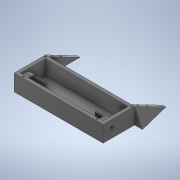
# Autodesk Inventor part: BodyWedgeV2
Saved by Autodesk Inventor 2020 (Build 240168000, 168)
## iProperties
Created: 2023-11-26
Part Number: BodyWedgeV2
Material: Thermoplastic Resin
Document SubType Name: Modeling
Designer: smz3rm
Density: 1.28 g/cm^3
Appearance: Smooth - Black
Mass: 160.779 g
Surface Area: 550.201 cm^2
Volume: 125.609 cm^3
Author: smz3rm
Autodesk Inventor part; units mm, degrees
ref_plane "YZ Plane" through (0, 0, 0) normal (1, 0, 0) x (0, 1, 0)
ref_plane "XZ Plane" through (0, 0, 0) normal (0, 1, 0) x (-1, 0, 0)
sketch "Sketch1" plane through (0, 0, 0) normal (0, 1, 0) x (-1, 0, 0)
  line L0 (85, 30) -> (-85, 30)
  line L1 (-85, 30) -> (-85, -30)
  line L2 (-85, -30) -> (85, -30)
  line L3 (85, -30) -> (85, 30)
  line L4 (85, 30) -> (-85, -30) construction
  line L5 (-85, 30) -> (85, -30) construction
  line L6 (0, -42) -> (0, 42) projected
  point P0 (0, 0)
  point P1 (-100, -30)
  point P2 (-85, -27)
  dimension "d0" = 170
  dimension "d1" = 60
  dimension "d32" = 15
  constraints: 12 end point, 2 midpoint, 2 parallel, 2 point on line, 1 horizontal, 1 perpendicular
  measures "d0" distance of L2.end L1.end
  measures "d1" distance of L1.end L0.end
  measures "d32" distance of L1.end point (-100, -30)
extrude "Extrusion1" add sketch "Sketch1" along normal blind 3
sketch "Sketch2" plane through (0, 3, 0) normal (0, 1, 0) x (1, 0, 0)
  line L0 (-85, 30) -> (-85, -30) projected
  line L1 (-85, -30) -> (85, -30) projected
  line L2 (85, -30) -> (85, 30) projected
  line L3 (79, -24) -> (-79, -24)
  line L4 (-79, -24) -> (-79, 24)
  line L5 (-79, 24) -> (79, 24)
  line L6 (79, 24) -> (79, -24)
  line L7 (79, -24) -> (-79, 24) construction
  line L8 (-79, -24) -> (79, 24) construction
  line L9 (85, 30) -> (-85, 30) projected
  point P0 (0, 0)
  dimension "d36" = 158
  dimension "d37" = 48
  constraints: 12 end point, 2 midpoint, 2 parallel, 1 horizontal, 1 perpendicular
  measures "d36" distance of L4.end L5.end
  measures "d37" distance between parallel lines of L5 L3
extrude "Extrusion2" add sketch "Sketch2" along normal blind 28
sketch "Sketch7" plane through (-79, 3, 24) normal (1, 0, 0) x (0, 0, -1)
  circle A0 centre (10, 14) radius 8
  line L0 (54, -3) -> (-6, -3) projected
  circle A1 centre (10, 14) radius 10
  line L1 (0, 14) -> (0, 0)
  line L2 (0, 14) -> (20, 14)
  line L3 (20, 14) -> (20, 0)
  line L4 (-6, -3) -> (-6, 28) projected
  line L5 (0, 0) -> (20, 0)
  line L6 (10, 24) -> (0, 24)
  line L7 (0, 0) -> (0, 28) projected
  line L8 (0, 14) -> (0, 24)
  point P0 (24, -3)
  point P1 (54, -3)
  dimension "MotorDiameter" = 16
  dimension "d18" = 17
  dimension "d20" = 2
  dimension "d40" = 20
  dimension "d62" = 10
  constraints: 12 end point, 3 horizontal, 3 point on circle, 2 centre point, 2 vertical, 1 perpendicular, 1 point on line
  measures "MotorDiameter" diameter of A0
  measures "d18" distance from line of L0 A0.centre
  measures "d20" radial gap between concentric circles of A0 A1
  measures "d40" distance between parallel lines of L3 L1
  measures "d62" distance of L6.start L6.end
extrude "Extrusion5" add sketch "Sketch7" along normal blind 11.25 contours L2 A1 A0 | A0 L2 A1 | L3 L5 L1 A1 | L7 L6 A1
sketch "Sketch8" plane through (-67.75, 3, 24) normal (1, 0, 0) x (0, 0, -1)
  arc A0 (20, 14) -> (10, 24) centre (10, 14) ccw projected
  circle A1 centre (10, 14) radius 8 projected
  line L0 (0, 0) -> (0, 24) projected
  line L1 (20, 0) -> (0, 0) projected
  line L2 (20, 0) -> (20, 14) projected
  circle A2 centre (10, 14) radius 7.75
  line L3 (10, 24) -> (0, 24) projected
  line L4 (0, 0) -> (0, 24) projected
  line L5 (4, 9.0946) -> (4, 19.2915)
  line L6 (10, 24) -> (0, 24) projected
  line L7 (16, 9.0946) -> (16, 19.2915)
  line L8 (16, 19.2915) -> (18.4853, 19.2915)
  arc A3 (20, 14) -> (10, 24) centre (10, 14) ccw projected
  line L9 (4, 19.2915) -> (0, 19.2915)
  point P0 (24, -3)
  point P1 (4, 27)
  point P2 (4, 18.9054)
  point P3 (16, 18.9054)
  dimension "d55" = 15.5
  dimension "d63" = 12
  dimension "d64" = 6
  constraints: 8 end point, 6 point on circle, 2 coincident, 2 perpendicular, 2 point on line, 1 centre point, 1 horizontal, 1 vertical
  measures "d55" diameter of A2
  measures "d63" distance between parallel lines of L7 L5
  measures "d64" distance from line of L5 point (10, 14)
extrude "Extrusion6" add sketch "Sketch8" along normal blind 20 contours L2 L1 L0 L9 A1 L8 A0 | A1 L5 A2 L7 | A2 L7 | L5 A2 picked at (9.114, 6.2488)
sketch "Sketch9" plane through (-79, 20, 20) normal (1, 0, 0) x (0, 0, -1)
  circle A0 centre (6, -3) radius 3.5
  line L0 (50, -20) -> (-10, -20) projected
  line L1 (-10, -20) -> (-10, 11) projected
  point P0 (20, -20)
  point P1 (44, -20)
  dimension "d27" = 7
  dimension "d28" = 17
  dimension "d41" = 16
  constraints: 1 centre point
  measures "d27" diameter of A0
  measures "d28" distance from line of L0 A0.centre
  measures "d41" distance from line of L1 A0.centre
extrude "Extrusion7" cut sketch "Sketch9" against normal up to surface (6 mm away)
mirror "Mirror2" about plane through (0, 0, 0) normal (1, 0, 0) of "Extrusion7", "Extrusion6", "Extrusion5"
sketch "Sketch15" plane through (85, 0, 30) normal (1, 0, 0) x (0, 0, -1)
  line L0 (60, 31) -> (0, 31) projected
  line L1 (60, 31) -> (120, 0)
  line L2 (120, 0) -> (60, 0)
  circle A0 centre (16, 17) radius 3.5 projected
  line L3 (0, 0) -> (60, 0) projected
  line L4 (60, 0) -> (60, 31) projected
  line L5 (0, 31) -> (60, 31) projected
  line L6 (0, 0) -> (0, 31) projected
  point P0 (30, 0)
  dimension "d67" = 60
  constraints: 4 end point, 1 parallel
  measures "d67" distance of L2.end L1.end
extrude "Extrusion12" add sketch "Sketch15" against normal blind 6 contours L1 L2 L4
mirror "Mirror5" about plane through (0, 0, 0) normal (1, 0, 0) of "Extrusion12"
sketch "Sketch16" plane through (79, 0, -30) normal (0, 0, -1) x (-1, 0, 0)
  line L0 (-6, 0) -> (-6, 31) projected
  line L1 (-6, 0) -> (0, 0) projected
  line L2 (0, 31) -> (0, 0) projected
  line L3 (-6, 31) -> (0, 31) projected
  line L4 (200.8, 0) -> (-56.8, 0) projected
  line L5 (-6, 31) -> (-21, 0)
  line L6 (-6, 0) -> (-21, 0)
  point P0 (79, 0)
  dimension "SideOffset" = 15
  constraints: 4 end point, 1 collinear, 1 point on line
  measures "SideOffset" distance from line of L0 L5.end
extrude "Extrusion13" add sketch "Sketch16" along normal blind 60 contours L4 L5 L0
ref_plane "Work Plane2" through (85, 31, -30) normal (-0.8782, -0.4249, 0.2195) x (0, -0.459, -0.8884)
sketch "Sketch19" plane through (85, 31, -30) normal (-0.8782, -0.4249, 0.2195) x (0, -0.459, -0.8884)
  line L0 (-86.7961, -100.9494) -> (167.9591, -100.9494)
  line L1 (167.9591, -100.9494) -> (167.9591, 132.7149)
  line L2 (167.9591, 132.7149) -> (-86.7961, 132.7149)
  line L3 (-86.7961, 132.7149) -> (-86.7961, -100.9494)
  point P0 (-12.4232, -4.3756)
  constraints: 8 end point, 2 parallel, 1 horizontal, 1 perpendicular
extrude "Extrusion14" cut sketch "Sketch19" against normal blind 60
mirror "Mirror8" about plane through (0, 0, 0) normal (1, 0, 0) of "Extrusion13", "Extrusion14"
sketch "Sketch20" plane through (79, 0, -90) normal (0, 0.8884, -0.459) x (1, 0, 0)
  line L0 (6, 0) -> (6, -67.5352) projected
  line L1 (6, 0) -> (0, 0) projected
  line L2 (0, -67.5352) -> (0, 0) projected
  line L3 (6, -67.5352) -> (0, -67.5352) projected
  line L4 (-164, 0) -> (-164, -67.5352) projected
  line L5 (-158, -67.5352) -> (-164, -67.5352) projected
  line L6 (-158, -67.5352) -> (-158, 0) projected
  line L7 (-164, 0) -> (-158, 0) projected
  circle A0 centre (3, -57.5352) radius 1.45
  line L8 (6, -67.5352) -> (0, -67.5352) projected
  line L9 (3, -67.5352) -> (3, 0)
  circle A1 centre (3, -37.5352) radius 1.45
  line L10 (-79, 24.6917) -> (-79, -148.1499) projected
  circle A2 centre (-161, -57.5352) radius 1.45
  circle A3 centre (-161, -37.5352) radius 1.45
  point P0 (-79, -79.9583)
  dimension "d75" = 2.9
  dimension "d76" = 10
  dimension "d77" = 2.9
  dimension "d78" = 20
  constraints: 4 centre point, 2 end point, 2 midpoint, 2 point on line, 2 symmetric about line, 2 other
  measures "d75" diameter of A0
  measures "d76" distance from line of L3 A0.centre
  measures "d77" diameter of A1
  measures "d78" distance of A1.centre A0.centre
extrude "Extrusion15" cut sketch "Sketch20" against normal blind 6.5 contours A1 L9 | L9 A1 | L9 A0 | A0 L9 | A2 | A3
sketch "Sketch21" plane through (0, 31, 0) normal (0, 1, 0) x (1, 0, 0)
  line L0 (85, -30) -> (85, 30) projected
  line L1 (85, 30) -> (79, 30) projected
  line L2 (79, 30) -> (-79, 30) projected
  line L3 (-79, 30) -> (-85, 30) projected
  line L4 (-85, 30) -> (-85, -30) projected
  line L5 (-85, -30) -> (85, -30) projected
  line L6 (79, 24) -> (79, -24) projected
  line L7 (79, -24) -> (-79, -24) projected
  line L8 (-79, -24) -> (-79, 24) projected
  line L9 (-79, 24) -> (79, 24) projected
  line L10 (82, -30) -> (82, 30)
  line L11 (85, 30) -> (79, 30) projected
  line L12 (85, -30) -> (85, 30) projected
  line L13 (85, -27) -> (-85, -27)
  line L14 (-85, 30) -> (-85, -30) projected
  line L15 (85, 27) -> (-85, 27)
  circle A0 centre (82, 27) radius 1.45
  line L16 (0, 42) -> (0, -42) projected
  circle A1 centre (-82, 27) radius 1.45
  circle A2 centre (70, -27) radius 1.45
  circle A3 centre (-70, -27) radius 1.45
  point P0 (0, 0)
  dimension "d82" = 3
  dimension "d83" = 3
  dimension "d84" = 3
  dimension "d85" = 2.9
  dimension "d86" = 2.9
  dimension "d87" = 15
  constraints: 8 point on line, 6 end point, 4 centre point, 2 perpendicular, 2 symmetric about line, 1 midpoint, 2 other
  measures "d82" distance of L0.start L13.start
  measures "d83" distance of L0.start L10.start
  measures "d84" distance of L0.end L15.start
  measures "d85" diameter of A0
  measures "d86" diameter of A2
  measures "d87" distance from line of L0 A2.centre
extrude "Extrusion16" cut sketch "Sketch21" against normal blind 6.5 contours A0 L10 L15 | L15 L10 A0 | A0 L15 L10 | A2 L13 | L13 A2 | L15 A0 L10 | A3 L13 | L13 A3 | A1 L15 | L15 A1
ref_plane "Work Plane3" through (-85, 31, -30) normal (-0.8782, 0.4249, -0.2195) x (0, -0.459, -0.8884)
equation "\"d0\" = Width"
equation "\"d1\" = Length"
equation "\"d32\" = -0.5 * Width + 0.5 * FullWidth"
equation "\"d2\" = BaseWallThickness"
equation "\"d36\" = Width - 2 * SideWallThickness"
equation "\"d37\" = Length - 2 * SideWallThickness"
equation "\"d5\" = Height - 2 * BaseWallThickness"
equation "\"d18\" = DriveMotorHeight"
equation "\"d20\" = DriveMotorMountThickness"
equation "\"d28\" = DriveMotorHeight"
equation "\"d41\" = SideWallThickness + DriveMotorMountThickness + 0.5 * MotorDiameter"
equation "\"d67\" = WedgeLength"
equation "\"d68\" = SideWallThickness"
equation "\"SideOffset\" = SideTriangleWidth"
equation "\"d71\" = WedgeLength"
equation "\"d73\" = WedgeLength"
equation "\"d75\" = ScrewHoleDia"
equation "\"d77\" = ScrewHoleDia"
equation "\"d79\" = ScrewDepth"
equation "\"d82\" = 0.5 * SideWallThickness"
equation "\"d83\" = 0.5 * SideWallThickness"
equation "\"d84\" = 0.5 * SideWallThickness"
equation "\"d85\" = ScrewHoleDia"
equation "\"d86\" = ScrewHoleDia"
equation "\"d88\" = ScrewDepth"
equation "\"SideWallThickness\" = 6"
equation "\"BaseWallThickness\" = 3"
equation "\"Width\" = 170"
equation "\"Length\" = 60"
equation "\"Height\" = 34"
equation "\"DriveMotorHeight\" = 17"
equation "\"DriveMotorMountThickness\" = 2"
equation "\"WedgeLength\" = 60"
equation "\"SideTriangleWidth\" = 15"
equation "\"ScrewHoleDia\" = 2.9"
equation "\"ScrewDepth\" = 6.5"
equation "\"FullWidth\" = 200"
body "Solid1"
